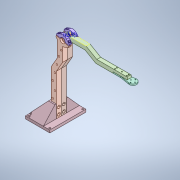
# Autodesk Inventor part: Луч
Saved by Autodesk Inventor 2021.2 (Build 252289000, 289)
## iProperties
Created: 2024-10-23
Part Number: Луч
Material: Типовые
Document SubType Name: Modeling
Designer: barko
Density: 1 g/cm^3
Appearance: По умолчанию
Author: barko
Autodesk Inventor part; units mm, degrees
ref_plane "XZ Plane" through (0, 0, 0) normal (0, 1, 0) x (-1, 0, 0)
ref_plane "XY Plane" through (0, 0, 0) normal (0, 0, 1) x (1, 0, 0)
sketch "Эскиз1" plane through (0, 0, 0) normal (0, 0, 1) x (1, 0, 0)
  circle A0 centre (0, 0) radius 5 construction
  line L0 (381, 7) -> (127, 7) construction
  line L1 (127, 7) -> (127, 17) construction
  line L2 (127, 17) -> (381, 17) construction
  line L3 (381, 17) -> (381, 7) construction
  line L4 (381, 7) -> (127, 17) construction
  line L5 (127, 7) -> (381, 17) construction
  arc A1 (0, 15) -> (14.8661, -2) centre (0, 0) ccw
  arc A2 (5.5, 0) -> (5.1235, -2) centre (0, 0) ccw
  line L6 (268, -19) -> (240, -19) construction
  line L7 (240, -19) -> (240, 7) construction
  line L8 (240, 7) -> (268, 7) construction
  line L9 (268, 7) -> (268, -19) construction
  line L10 (268, -19) -> (240, 7) construction
  line L11 (240, -19) -> (268, 7) construction
  line L12 (0, 15) -> (79.4308, 15)
  line L13 (79.4308, 15) -> (121, -9)
  line L14 (121, -9) -> (254, -9)
  line L15 (254, -9) -> (254, -24)
  line L16 (254, -24) -> (116.9808, -24)
  line L17 (116.9808, -24) -> (75.4115, 0)
  line L18 (75.4115, 0) -> (5.5, 0)
  line L19 (10, 15) -> (10, -15) construction
  line L20 (12.5, -6) -> (7.5, -6) construction
  line L21 (7.5, -6) -> (7.5, 13) construction
  line L22 (7.5, 13) -> (12.5, 13) construction
  line L23 (12.5, 13) -> (12.5, -6) construction
  line L24 (12.5, -6) -> (7.5, 13) construction
  line L25 (7.5, -6) -> (12.5, 13) construction
  line L26 (15, 13) -> (5, 13) construction
  line L27 (5, 13) -> (5, 16) construction
  line L28 (5, 16) -> (15, 16) construction
  line L29 (15, 16) -> (15, 13) construction
  line L30 (15, 13) -> (5, 16) construction
  line L31 (5, 13) -> (15, 16) construction
  line L32 (15, -15) -> (5, -15) construction
  line L33 (5, -15) -> (5, -6) construction
  line L34 (5, -6) -> (15, -6) construction
  line L35 (15, -6) -> (15, -15) construction
  line L36 (15, -15) -> (5, -6) construction
  line L37 (5, -15) -> (15, -6) construction
  line L38 (14.8661, -2) -> (5.1235, -2)
  line L39 (14.8661, -2) -> (15.8661, -2)
  line L40 (15.8661, -2) -> (15.8661, -12)
  line L41 (15.8661, -12) -> (9, -12)
  point P0 (254, 12)
  point P1 (254, -6)
  point P2 (254, -6)
  point P3 (254, 12)
  point P4 (10, 3.5)
  point P5 (10, 14.5)
  point P6 (10, -10.5)
  point P7 (10, -6)
  point P8 (10, 13)
  point P9 (13.7477, -6)
  dimension "d0" = 10
  dimension "d1" = 10
  dimension "d2" = 254
  dimension "d3" = 254
  dimension "d4" = 7
  dimension "d6" = 26
  dimension "d8" = 28
  dimension "d9" = 15
  dimension "d10" = 15
  dimension "d11" = 15
  dimension "d12" = 5
  dimension "d14" = 0.5
  dimension "d17" = 0
  dimension "d21" = 5
  dimension "d23" = 2
  dimension "d24" = 10
  dimension "d25" = 10
  dimension "d27" = 1
  dimension "d29" = 30
  dimension "d30" = 6
  dimension "d31" = 0
  dimension "d48" = 24
  dimension "d78" = 2
  dimension "d79" = 2
  dimension "d80" = 4
  dimension "d115" = 0
  dimension "d237" = 10
  dimension "d245" = 1
  constraints: 84 end point, 17 midpoint, 12 parallel, 10 horizontal, 7 perpendicular, 7 point on circle, 6 point on line, 3 centre point, 3 coincident, 2 vertical, 1 tangent, 1 vertical alignment
  measures "d0" diameter of A0
  measures "d1" distance of L0.end L1.end
  measures "d2" distance of L1.end L2.end
  measures "d3" horizontal distance of point (254, 12) point (0, 0)
  measures "d4" distance from line of point (0, 0) L0
  measures "d6" distance of L8.end L6.start
  measures "d8" distance of L6.start L6.end
  measures "d9" distance between parallel lines of L12 L18
  measures "d10" distance between parallel lines of L13 L17
  measures "d11" distance between parallel lines of L16 L14
  measures "d12" distance between parallel lines of L6 L16
  measures "d14" radial gap between concentric circles of A0 A2
  measures "d17" distance from line of point (0, 0) L18
  measures "d21" distance of L21.end L22.end
  measures "d23" distance between parallel lines of L12 L26
  measures "d24" distance of L32.start L32.end
  measures "d25" distance of L27.end L28.end
  measures "d27" distance between parallel lines of L12 L28
  measures "d29" angle of L12 L13
  measures "d30" distance from line of L1 L13.end
  measures "d31" distance from line of point (254, -6) L15
  measures "d48" distance between parallel lines of L18 L16
  measures "d78" distance between parallel lines of L18 L38
  measures "d79" distance edge to line of A2 L21
  measures "d80" distance between parallel lines of L38 L20
  measures "d115" distance edge to line of A1 L32
  measures "d237" distance of L39.end L40.end
  measures "d245" distance of L38.start L39.end
extrude "Выдавливание1" add sketch "Эскиз1" along normal mid plane 15
sketch "Эскиз2" plane through (116.9808, -24, 7.5) normal (0, -1, 0) x (1, 0, 0)
  circle A0 centre (137.0192, -7.5) radius 14
  circle A1 centre (137.0192, -7.5) radius 16
  line L0 (0, 0) -> (137.0192, 0) construction
  line L1 (137.0192, -15) -> (0, -15) construction
  line L2 (97.0192, 0) -> (134.7082, 6.3079)
  line L3 (4.0192, -15) -> (137.0192, -15) construction
  line L4 (97.0192, -15) -> (134.7082, -21.3079)
  line L5 (97.0192, 0) -> (97.0192, -15)
  line L6 (97.0192, 0) -> (67.0192, 0)
  line L7 (67.0192, 0) -> (67.0192, -15)
  line L8 (67.0192, -15) -> (97.0192, -15)
  point P0 (-116.9808, -7.5)
  point P1 (137.0192, -7.5)
  dimension "d34" = 28
  dimension "d35" = 2
  dimension "d40" = 40
  dimension "d75" = 30
  constraints: 12 end point, 4 point on line, 2 centre point, 2 coincident, 2 perpendicular, 2 point on circle, 2 tangent, 1 vertical
  measures "d34" diameter of A0
  measures "d35" radial gap between concentric circles of A0 A1
  measures "d40" horizontal distance of A0.centre L2.start
  measures "d75" distance between parallel lines of L5 L7
extrude "Выдавливание2" add sketch "Эскиз2" against normal blind 5 separate body contours A0 | A0 L4 A1 L2 | A1 L4 L5 L2 | L5 L8 L7 L6 picked at (121.8202, -8.6894)
extrude "Выдавливание3" cut sketch "Эскиз2" against normal up to surface (10 mm away) from surface at -5 contours A0 | A0 L2 A1 L4 | A0 L4 A1 L2 bodies 1
extrude "Выдавливание11" cut sketch "Эскиз2" against normal up to surface (5 mm away) from surface at 0 contours A0 | A0 L4 A1 L2 | A1 L4 L5 L2 | L5 L8 L7 L6 picked at (121.8202, -8.6894) bodies 1
sketch "Эскиз3" plane through (0, 0, 0) normal (0, 0, 1) x (1, 0, 0)
  line L0 (-250, -275) -> (250, -275) construction
  circle A0 centre (0, 0) radius 381 construction
  circle A1 centre (0, 0) radius 9.5 construction
  arc A2 (-9.9382, 1.11) -> (9.1617, -4.0078) centre (0, 0) ccw
  arc A3 (-19.6523, 3.7129) -> (18.8759, -6.6107) centre (0, 0) ccw
  line L1 (-20, 0) -> (-20, -7.0273) construction
  line L2 (0, -73.4115) -> (0, -20)
  line L3 (251.689, -24) -> (268, -24) construction
  line L4 (116.9808, -24) -> (75.4115, 0) construction
  circle A4 centre (0, 0) radius 75.4115 construction
  arc A5 (5.5, 0) -> (5.1235, -2) centre (0, 0) ccw construction
  line L5 (254, -24) -> (116.9808, -24) construction
  circle A6 centre (0, 0) radius 119.4173 construction
  circle A7 centre (0, 0) radius 269.0725 construction
  line L6 (0, -73.4115) -> (-24, -114.9808)
  line L7 (-24, -114.9808) -> (-24, -275)
  line L8 (-20, -68.0526) -> (-44, -109.6218)
  line L9 (-44, -109.6218) -> (-44, -275)
  line L10 (-44, -275) -> (-24, -275)
  line L11 (-19.6523, 3.7129) -> (18.8759, -6.6107)
  line L12 (-18.8759, 6.6107) -> (19.6523, -3.7129)
  line L13 (-533.4, 0) -> (533.4, 0) construction
  arc A8 (19.6523, -3.7129) -> (-18.8759, 6.6107) centre (0, 0) ccw
  arc A9 (-9.1617, 4.0078) -> (-9.9382, 1.11) centre (0, 0) ccw
  arc A10 (9.1617, -4.0078) -> (9.9382, -1.11) centre (0, 0) ccw
  arc A11 (9.9382, -1.11) -> (-9.1617, 4.0078) centre (0, 0) ccw
  circle A12 centre (0, 0) radius 6.5
  line L14 (-18.8759, 6.6107) -> (-23.7055, 7.9048)
  line L15 (-22.4114, 12.7344) -> (-16.5875, 11.1739)
  line L16 (-19.6523, 3.7129) -> (-24.482, 5.007)
  line L17 (-25.7761, 0.1774) -> (-19.9521, -1.3831)
  line L18 (-23.7055, 7.9048) -> (-22.4114, 12.7344)
  line L19 (-24.482, 5.007) -> (-25.7761, 0.1774)
  line L20 (-22.4114, 12.7344) -> (-7.2587, 18.6363)
  line L21 (-25.7761, 0.1774) -> (-15.6044, -12.5101)
  line L22 (19.6523, -3.7129) -> (24.482, -5.007)
  line L23 (24.482, -5.007) -> (25.7761, -0.1774)
  line L24 (25.7761, -0.1774) -> (15.6044, 12.5101)
  line L25 (25.7761, -0.1774) -> (19.9521, 1.3831)
  line L26 (18.8759, -6.6107) -> (23.7055, -7.9048)
  line L27 (23.7055, -7.9048) -> (22.4114, -12.7344)
  line L28 (22.4114, -12.7344) -> (16.5875, -11.1739)
  line L29 (22.4114, -12.7344) -> (7.2587, -18.6363)
  line L30 (-20, -7.0273) -> (-20, -68.0526)
  arc A13 (-20, -15) -> (0, -25) centre (0, 0) ccw
  arc A14 (0, 15) -> (9, -12) centre (0, 0) ccw construction
  line L31 (0, 0) -> (66.16, -375.2118) construction
  point P0 (0, -275)
  point P1 (0, -75.4115)
  point P2 (0, -119.4173)
  point P3 (5.7208, -3.0858)
  point P4 (-6.4973, 0.188)
  point P5 (-5.7208, 3.0858)
  point P6 (6.4973, -0.188)
  point P7 (-20, -1.3703)
  dimension "d107" = 381
  dimension "d108" = 538.145
  dimension "d43" = 275
  dimension "d44" = 500
  dimension "d45" = 19
  dimension "d46" = 0.5
  dimension "d47" = 20
  dimension "d49" = 30
  dimension "d50" = 24
  dimension "d53" = 20
  dimension "d54" = 20
  dimension "d56" = 3
  dimension "d57" = 1.5
  dimension "d58" = 15
  dimension "d59" = 3
  dimension "d93" = 5
  dimension "d94" = 5
  dimension "d95" = 5
  dimension "d102" = 5
  dimension "d105" = 80
  dimension "d246" = 2
  constraints: 56 end point, 20 point on circle, 10 centre point, 10 point on line, 9 coincident, 8 parallel, 7 perpendicular, 4 equal length, 4 vertical, 3 vertical alignment, 2 collinear, 2 horizontal, 2 tangent, 1 midpoint, 19 other
  measures "d43" distance from line of L0 point (0, 0)
  measures "d44" distance of L0.start L0.end
  measures "d45" diameter of A1
  measures "d46" radial gap between concentric circles of A1 A2
  measures "d47" distance between parallel lines of L2 L1
  measures "d49" angle of L2 L6
  measures "d50" distance between parallel lines of L2 L7
  measures "d53" distance between parallel lines of L6 L8
  measures "d54" distance between parallel lines of L7 L9
  measures "d56" distance between parallel lines of L12 L11
  measures "d57" distance from line of point (0, 0) L12
  measures "d58" angle of L13 L11
  measures "d59" radial gap between concentric circles of A12 A1
  measures "d93" distance between parallel lines of L15 L14
  measures "d94" distance between parallel lines of L17 L16
  measures "d95" distance of L12.start L14.end
  measures "d105" angle of L13 L31
  measures "d246" distance of A4.end L2.start
ref_plane "РабПлоскость1" through (0, 0, 9.5) normal (0, 0, 1) x (1, 0, 0)
extrude "Выдавливание12" add sketch "Эскиз3" along normal blind 3 from surface at 9.5 separate body contours L11 A12 A2 | A2 L11 A3
extrude "Выдавливание13" add sketch "Эскиз3" along normal blind 7 from surface at 12.5 contours A2 L11 A3 bodies 3
extrude "Выдавливание17" add sketch "Эскиз3" along normal up to surface (10 mm away) from surface at 9.5 contours A3 L17 L19 L16 | L26 L27 L28 A3 | A3 L21 L17 | L28 L29 A3 bodies 3
extrude "Выдавливание15" add sketch "Эскиз3" along normal up to surface (3 mm away) from surface at 9.5 separate body contours A11 L12 A12 | L12 A8 A11
extrude "Выдавливание16" add sketch "Эскиз3" along normal up to surface (7 mm away) from surface at 12.5 contours L12 A8 A11 bodies 4
extrude "Выдавливание18" add sketch "Эскиз3" along normal up to surface (10 mm away) from surface at 9.5 contours L14 L18 L15 A8 | A8 L25 L23 L22 | L15 L20 A8 | A8 L24 L25 bodies 4
extrude "Выдавливание19" add sketch "Эскиз3" along normal up to surface (10 mm away) from surface at 9.5 contours A3 L2 A13 L30 L21 | L2 L6 L7 L10 L9 L8 L30 A13 bodies 3
extrude "Выдавливание20" add sketch "Эскиз3" along normal up to surface (9.5 mm away) contours L2 L6 L7 L10 L9 L8 L30 A13 bodies 3
sketch "Эскиз4" plane through (0, 0, 0) normal (0, 0, 1) x (1, 0, 0)
  circle A0 centre (0, 0) radius 269.0725 construction
  circle A1 centre (0, 0) radius 119.4173 construction
  line L0 (184, -24) -> (116.9808, -24) construction
  line L1 (268, -24) -> (116.9808, -24) construction
  line L2 (116.9808, -24) -> (0, 0) construction
  arc A2 (5.5, 0) -> (5.1235, -2) centre (0, 0) ccw construction
  line L3 (-3.3219, -119.3711) -> (22.9023, -268.096) construction
  line L4 (-3.3219, -119.3711) -> (0, 0) construction
  line L5 (-44, -109.6218) -> (-44, -275) construction
  line L6 (-44, -275) -> (-24, -275) construction
  line L7 (-24, -275) -> (-24, -114.9808) construction
  line L8 (381, 7) -> (127, 7) construction
  line L9 (28.947, -123.855) -> (73.0536, -373.9962) construction
  arc A3 (28.947, -123.855) -> (127, 7) centre (0, 0) ccw construction
  line L10 (1, -275) -> (-94, -275)
  line L11 (-94, -275) -> (-94, -285)
  line L12 (-94, -285) -> (1, -285)
  line L13 (1, -285) -> (1, -275)
  line L14 (-44, -275) -> (-44, -109.6218) construction
  line L15 (-24, -275) -> (-44, -275) construction
  dimension "d109" = 168.406
  dimension "d110" = 0
  dimension "d112" = 149.6551
  dimension "d113" = 168.406
  dimension "d114" = 80
  dimension "d116" = 31
  dimension "d117" = 31
  dimension "d118" = 10
  dimension "d119" = 25
  dimension "d120" = 50
  constraints: 18 end point, 6 point on circle, 3 parallel, 1 centre point, 1 coincident, 1 collinear, 1 equal length, 1 horizontal, 1 perpendicular, 1 point on line
  measures "d109" angle of L2 L1
  measures "d110" distance between parallel lines of L0 L1
  measures "d112" radial gap between concentric circles of A1 A0
  measures "d113" angle of L4 L3
  measures "d114" angle of L2 L4
  measures "d116" distance between parallel lines of L0 L8
  measures "d117" distance between parallel lines of L3 L9
  measures "d118" distance of L12.end L10.start
  measures "d119" distance between parallel lines of L7 L13
  measures "d120" distance between parallel lines of L5 L11
ref_plane "РабПлоскость2" through (-44, -275, 69.5) normal (0, 0, 1) x (1, 0, 0)
extrude "Выдавливание24" add sketch "Эскиз4" along normal blind 70 separate body
ref_plane "РабПлоскость3" through (-94, -225, 0) normal (0, 1, 0) x (1, 0, 0)
sketch "Эскиз6" plane through (-94, -225, 0) normal (0, 1, 0) x (1, 0, 0)
  line L0 (103.1617, -19.5) -> (117.7055, -19.5) construction
  line L1 (84.0618, -19.5) -> (103.1617, -19.5) construction
  line L2 (69.518, -19.5) -> (84.0618, -19.5) construction
  line L3 (68.2239, -19.5) -> (69.518, -19.5) construction
  line L4 (74, -19.5) -> (68.2239, -19.5) construction
  line L5 (50, -19.5) -> (74, -19.5) construction
  line L6 (70, -19.5) -> (50, -19.5) construction
  line L7 (94, -19.5) -> (70, -19.5) construction
  line L8 (101.2587, -19.5) -> (94, -19.5) construction
  line L9 (116.4114, -19.5) -> (101.2587, -19.5) construction
  line L10 (117.7055, -19.5) -> (116.4114, -19.5) construction
  line L11 (50, 0) -> (50, -19.5) construction
  line L12 (50, 0) -> (50, -19.5) construction
  line L13 (70, 0) -> (94, 0) construction
  line L14 (50, 0) -> (70, 0) construction
  line L15 (74, 0) -> (50, 0) construction
  line L16 (94, 0) -> (74, 0) construction
  line L17 (70, 0) -> (70, -19.5) construction
  line L18 (70, 0) -> (70, -19.5) construction
  line L19 (95, 0) -> (95, -70) construction
  line L20 (95, 0) -> (0, 0) construction
  line L21 (0, 0) -> (0, -70) construction
  line L22 (95, 0) -> (0, 0) construction
  line L23 (49.5, 0) -> (49.5, -20)
  line L24 (49.5, -20) -> (70, -20)
  line L25 (70, 0) -> (70, -19.5) construction
  line L26 (70, -20) -> (70, 0)
  line L27 (70, 0) -> (49.5, 0)
  line L28 (49.5, 0) -> (44.5, 0)
  line L29 (44.5, 0) -> (44.5, -25)
  line L30 (44.5, -25) -> (70, -25)
  line L31 (70, -25) -> (70, -20)
  line L32 (95, -70) -> (0, -70) projected
  point P0 (94, 0)
  dimension "d136" = 0.5
  dimension "d137" = 0.5
  dimension "d148" = 5
  dimension "d149" = 5
  constraints: 16 end point, 4 perpendicular, 2 vertical, 1 collinear, 3 other
  measures "d136" distance between parallel lines of L11 L23
  measures "d137" distance between parallel lines of L6 L24
  measures "d148" distance between parallel lines of L23 L29
  measures "d149" distance between parallel lines of L24 L30
sketch "Эскиз7" plane through (-94, -275, 0) normal (0, 1, 0) x (1, 0, 0)
  line L0 (95, 0) -> (0, 0) construction
  line L1 (70, 0) -> (70, -19.5) construction
  line L2 (0, 0) -> (70, 0)
  line L3 (70, 0) -> (70, -70)
  line L4 (0, 0) -> (0, -70) construction
  line L5 (0, 0) -> (0, -70) construction
  line L6 (0, 0) -> (0, -70)
  line L7 (0, -70) -> (70, -70)
  line L8 (95, -70) -> (0, -70) construction
  point P0 (94, 0)
  dimension "d191" = 0
  constraints: 8 end point, 2 perpendicular, 1 horizontal, 1 vertical
  measures "d191" distance between parallel lines of L8 L7
loft "Лофт1" add profiles "Эскиз7", "Эскиз6" bodies 5
extrude "Выдавливание25" cut sketch "Эскиз6" against normal up to surface (50 mm away) contours L27 L26 L24 L23 bodies 5
ref_plane "РабПлоскость5" through (-49.5, -225, 25) normal (1, 0, 0) x (0, 1, 0)
sketch "Эскиз9" plane through (-24, -225, 25) normal (1, 0, 0) x (0, 1, 0)
  line L0 (-8.9378, -15.25) -> (-11.9689, -20.5)
  line L1 (-11.9689, -20.5) -> (-18.0311, -20.5)
  line L2 (-18.0311, -20.5) -> (-21.0622, -15.25)
  line L3 (-21.0622, -15.25) -> (-18.0311, -10)
  line L4 (-18.0311, -10) -> (-11.9689, -10)
  line L5 (-11.9689, -10) -> (-8.9378, -15.25)
  circle A0 centre (-15, -15.25) radius 5.25 construction
  line L6 (-50, -5.5) -> (115.3782, -5.5) construction
  line L7 (115.3782, -25) -> (-50, -25) construction
  line L8 (0, 0) -> (0, -25) construction
  line L9 (-11.2472, -15.25) -> (-13.1236, -18.5)
  line L10 (-13.1236, -18.5) -> (-16.8764, -18.5)
  line L11 (-16.8764, -18.5) -> (-18.7528, -15.25)
  line L12 (-18.7528, -15.25) -> (-16.8764, -12)
  line L13 (-16.8764, -12) -> (-13.1236, -12)
  line L14 (-13.1236, -12) -> (-11.2472, -15.25)
  circle A1 centre (-15, -15.25) radius 3.25 construction
  line L15 (0, -21.8122) -> (-15, -21.8122)
  arc A2 (-15, -8.6878) -> (-15, -21.8122) centre (-15, -15.25) ccw
  line L16 (-15, -8.6878) -> (0, -8.6878)
  line L17 (0, -21.8122) -> (0, -8.6878)
  circle A3 centre (-15, -15.25) radius 6.0622 construction
  line L18 (-15, -15.25) -> (-40, -15.25)
  line L19 (-36.2472, -15.25) -> (-38.1236, -18.5)
  circle A4 centre (-40, -15.25) radius 3.25 construction
  line L20 (-41.8764, -18.5) -> (-43.7528, -15.25)
  line L21 (-33.9378, -15.25) -> (-36.9689, -20.5)
  line L22 (-36.9689, -20.5) -> (-43.0311, -20.5)
  circle A5 centre (-40, -15.25) radius 5.25 construction
  line L23 (-43.0311, -20.5) -> (-46.0622, -15.25)
  circle A6 centre (-40, -15.25) radius 6.0622 construction
  line L24 (-43.0311, -10) -> (-36.9689, -10)
  line L25 (-36.9689, -10) -> (-33.9378, -15.25)
  line L26 (-41.8764, -12) -> (-38.1236, -12)
  line L27 (-38.1236, -12) -> (-36.2472, -15.25)
  line L28 (-46.0622, -15.25) -> (-43.0311, -10)
  line L29 (-38.1236, -18.5) -> (-41.8764, -18.5)
  line L30 (-43.7528, -15.25) -> (-41.8764, -12)
  line L31 (-15, -8.6878) -> (-40, -8.6878)
  line L32 (110.0192, -5.5) -> (-50, -5.5) construction
  line L33 (-40, -21.8122) -> (-15, -21.8122)
  arc A7 (-40, -8.6878) -> (-40, -21.8122) centre (-40, -15.25) ccw
  point P0 (225, -25)
  dimension "d145" = 10.5
  dimension "d146" = 19.5
  dimension "d147" = 9.75
  dimension "d152" = 15
  dimension "d153" = 6.5
  dimension "d161" = 0.5
  dimension "d166" = 25
  constraints: 60 end point, 12 coincident, 7 tangent, 6 centre point, 6 horizontal, 5 point on circle, 2 horizontal alignment, 2 parallel, 2 point on line, 1 collinear, 1 perpendicular, 62 other
  measures "d145" distance between parallel lines of L4 L1
  measures "d146" distance between parallel lines of L6 L7
  measures "d147" distance from line of L7 point (-15, -15.25)
  measures "d152" distance from line of point (-15, -15.25) L8
  measures "d153" diameter of A1
  measures "d166" distance of L9.start L19.start
extrude "Выдавливание27" cut sketch "Эскиз9" against normal blind 69.5 contours L9 L10 L11 L12 L13 L14 | L19 L29 L20 L30 L26 L27 bodies 3 5
extrude "Выдавливание28" cut sketch "Эскиз9" against normal blind 7 from surface at 0 contours L0 L1 L2 L3 L4 L5 | L19 L29 L20 L30 L26 L27 | L21 L22 L23 L28 L24 L25 bodies 3
ref_plane "РабПлоскость6" through (-55.5, -225, 25) normal (1, 0, 0) x (0, 1, 0)
ref_plane "РабПлоскость7" through (-75.5, -225, 25) normal (1, 0, 0) x (0, 1, 0)
extrude "Выдавливание26" cut sketch "Эскиз9" along normal blind 6 from surface at -31.5 contours L0 L1 L2 L3 L4 L5 | L9 L10 L11 L12 L13 L14 bodies 5
extrude "Выдавливание29" cut sketch "Эскиз9" against normal up to surface (38.5 mm away) from surface at -31.5 contours L0 L1 L2 L3 L4 L5 | L9 L10 L11 L12 L13 L14 | L15 A2 L16 L17 bodies 5
extrude "Выдавливание31" cut sketch "Эскиз9" along normal blind 5 from surface at -51.5 contours L21 L22 L23 L28 L24 L25 bodies 5
extrude "Выдавливание32" cut sketch "Эскиз9" against normal up to surface (18.5 mm away) from surface at -51.5 contours L15 A2 L16 L17 | L33 A7 L31 A2 | L19 L29 L20 L30 L26 L27 | L21 L22 L23 L28 L24 L25 bodies 5
sketch "Эскиз11" plane through (1, -275, 70) normal (0, 1, 0) x (1, 0, 0)
  line L0 (0, 70) -> (0, 0) construction
  line L1 (-95, 0) -> (0, 0) construction
  line L2 (0, 0) -> (-25, 0) construction
  line L3 (-25, 0) -> (-95, 0) construction
  line L4 (-95, 70) -> (-95, 0) construction
  line L5 (-95, 70) -> (-95, 0) construction
  line L6 (-95, 0) -> (0, 0) construction
  line L7 (-95, 0) -> (-95, 14.75)
  line L8 (-95, 70) -> (-95, 0) construction
  line L9 (-95, 14.75) -> (-88.75, 14.75)
  arc A0 (-80.25, 6.25) -> (-88.75, 14.75) centre (-88.75, 6.25) ccw
  line L10 (-80.25, 6.25) -> (-80.25, 0)
  line L11 (-95, 0) -> (-80.25, 0)
  circle A1 centre (-6.25, 6.25) radius 3.25
  circle A2 centre (-88.75, 6.25) radius 3.25
  circle A3 centre (-88.75, 6.25) radius 7.5 construction
  circle A4 centre (-88.75, 6.25) radius 5.5 construction
  point P0 (-1, 70)
  dimension "d196" = 6.5
  dimension "d197" = 3
  dimension "d199" = 3
  dimension "d200" = 3
  dimension "d201" = 3
  dimension "d202" = 11
  dimension "d203" = 15
  dimension "d204" = 1
  constraints: 8 end point, 5 centre point, 3 coincident, 2 point on circle, 2 point on line, 2 tangent, 1 collinear, 1 equal radius, 1 horizontal, 1 perpendicular
  measures "d196" diameter of A2
  measures "d197" distance edge to line of A2 L1
  measures "d199" distance edge to line of A1 L1
  measures "d200" distance edge to line of A1 L0
  measures "d201" distance edge to line of A2 L4
  measures "d202" diameter of A4
  measures "d203" diameter of A3
  measures "d204" radial gap between concentric circles of A3 A0
extrude "Выдавливание35" cut sketch "Эскиз11" against normal through all contours A1 | A2 bodies 5
extrude "Выдавливание36" cut sketch "Эскиз11" along normal up to next contours L7 L9 A0 L10 L11 | A2 bodies 5
ref_plane "РабПлоскость8" through (-6.1091, 1.6369, 9.5) normal (-0.258819, -0.9659258, 0) x (0.9659258, -0.258819, 0)
sketch "Эскиз12" plane through (-6.1091, 1.6369, 9.5) normal (-0.258819, -0.9659258, 0) x (0.9659258, -0.258819, 0)
  line L0 (-3.5623, 3) -> (-3.5623, 10) construction
  line L1 (-3.5623, 3) -> (-3.5623, 10) construction
  line L2 (16.2114, 3) -> (16.2114, 10) construction
  line L3 (16.2114, 10) -> (16.2114, 3) construction
  line L4 (-18.6191, 0) -> (-18.6191, 10) construction
  line L5 (31.2682, 0) -> (31.2682, 10) construction
  circle A0 centre (26.0182, 5) radius 2.25 construction
  circle A1 centre (-13.3691, 5) radius 2.25 construction
  line L6 (-5.5102, 10) -> (18.1593, 10) construction
  line L7 (-5.5102, 0) -> (18.1593, 0) construction
  line L8 (-18.6191, 0) -> (-5.5102, 0) construction
  line L9 (26.0182, 0.8431) -> (22.4182, 2.9215)
  line L10 (22.4182, 2.9215) -> (22.4182, 7.0785)
  line L11 (22.4182, 7.0785) -> (26.0182, 9.1569)
  line L12 (26.0182, 9.1569) -> (29.6182, 7.0785)
  line L13 (29.6182, 7.0785) -> (29.6182, 2.9215)
  line L14 (29.6182, 2.9215) -> (26.0182, 0.8431)
  line L15 (-13.3691, 0.8431) -> (-16.9691, 2.9215)
  line L16 (-16.9691, 2.9215) -> (-16.9691, 7.0785)
  line L17 (-16.9691, 7.0785) -> (-13.3691, 9.1569)
  line L18 (-13.3691, 9.1569) -> (-9.7691, 7.0785)
  line L19 (-9.7691, 7.0785) -> (-9.7691, 2.9215)
  line L20 (-9.7691, 2.9215) -> (-13.3691, 0.8431)
  circle A2 centre (-13.3691, 5) radius 4.1569 construction
  circle A3 centre (26.0182, 5) radius 4.1569 construction
  line L21 (26.0182, 2.4019) -> (23.7682, 3.701)
  line L22 (23.7682, 3.701) -> (23.7682, 6.299)
  line L23 (23.7682, 6.299) -> (26.0182, 7.5981)
  line L24 (26.0182, 7.5981) -> (28.2682, 6.299)
  line L25 (28.2682, 6.299) -> (28.2682, 3.701)
  line L26 (28.2682, 3.701) -> (26.0182, 2.4019)
  line L27 (-13.3691, 2.4019) -> (-15.6191, 3.701)
  line L28 (-15.6191, 3.701) -> (-15.6191, 6.299)
  line L29 (-15.6191, 6.299) -> (-13.3691, 7.5981)
  line L30 (-13.3691, 7.5981) -> (-11.1191, 6.299)
  line L31 (-11.1191, 6.299) -> (-11.1191, 3.701)
  line L32 (-11.1191, 3.701) -> (-13.3691, 2.4019)
  line L33 (-18.6191, 0) -> (-18.6191, 10) construction
  line L34 (-11.1752, 0) -> (-18.6191, 0) construction
  line L35 (31.2682, 0) -> (31.2682, 10) construction
  line L36 (16.2114, 10) -> (31.2682, 10) construction
  point P0 (6.3246, -9.5)
  dimension "d303" = 8.3138
  dimension "d304" = 8.3138
  dimension "d209" = 4.5
  dimension "d210" = 4.5
  dimension "d211" = 10
  dimension "d212" = 5
  dimension "d213" = 5
  dimension "d215" = 3
  dimension "d218" = 3
  dimension "d306" = 7.2
  constraints: 48 end point, 6 coincident, 4 parallel, 2 centre point, 2 tangent, 58 other
  measures "d209" diameter of A0
  measures "d210" diameter of A1
  measures "d211" distance between parallel lines of L6 L7
  measures "d212" distance from line of A0.centre L7
  measures "d213" distance from line of A1.centre L8
  measures "d215" distance edge to line of A0 L5
  measures "d218" distance edge to line of A1 L4
  measures "d306" distance between parallel lines of L19 L16
ref_plane "РабПлоскость9" through (-8.1796, -6.0905, 9.5) normal (-0.258819, -0.9659258, 0) x (0.9659258, -0.258819, 0)
extrude "Выдавливание39" cut sketch "Эскиз12" along normal blind 23 from surface at 8 contours L9 L10 L11 L12 L13 L14 | L15 L16 L17 L18 L19 L20 | L21 L22 L23 L24 L25 L26 | L27 L28 L29 L30 L31 L32 bodies 3
extrude "Выдавливание38" cut sketch "Эскиз12" along normal blind 14 contours L21 L22 L23 L24 L25 L26 | L27 L28 L29 L30 L31 L32 bodies 3
extrude "Выдавливание50" cut sketch "Эскиз12" against normal blind 33 contours L21 L22 L23 L24 L25 L26 | L27 L28 L29 L30 L31 L32 bodies 4
ref_plane "РабПлоскость10" through (-4.815, 6.4665, 9.5) normal (-0.258819, -0.9659258, 0) x (0.9659258, -0.258819, 0)
extrude "Выдавливание51" cut sketch "Эскиз12" against normal blind 33 from surface at -5 contours L9 L10 L11 L12 L13 L14 | L15 L16 L17 L18 L19 L20 | L21 L22 L23 L24 L25 L26 | L27 L28 L29 L30 L31 L32 bodies 4
sketch "Эскиз13" plane through (0, 15, 7.5) normal (0, 1, 0) x (1, 0, 0)
  line L0 (0, 0) -> (0, 15) construction
  line L1 (79.4308, 0) -> (0, 0) construction
  line L2 (79.4308, 15) -> (79.4308, 0) construction
  line L3 (0, 15) -> (79.4308, 15) construction
  line L4 (5.5, 15) -> (5.5, 0) construction
  circle A0 centre (9.05, 7.5) radius 2.05 construction
  line L5 (9.05, 3.3431) -> (5.45, 5.4215)
  line L6 (5.45, 5.4215) -> (5.45, 9.5785)
  line L7 (5.45, 9.5785) -> (9.05, 11.6569)
  line L8 (9.05, 11.6569) -> (12.65, 9.5785)
  line L9 (12.65, 9.5785) -> (12.65, 5.4215)
  line L10 (12.65, 5.4215) -> (9.05, 3.3431)
  line L11 (9.05, 5.1329) -> (7, 6.3164)
  line L12 (7, 6.3164) -> (7, 8.6836)
  line L13 (7, 8.6836) -> (9.05, 9.8671)
  line L14 (9.05, 9.8671) -> (11.1, 8.6836)
  line L15 (11.1, 8.6836) -> (11.1, 6.3164)
  line L16 (11.1, 6.3164) -> (9.05, 5.1329)
  line L17 (0, 15) -> (79.4308, 15) construction
  line L18 (15.8661, 15) -> (15.8661, 0) construction
  point P0 (0, 7.5)
  dimension "d226" = 4.1
  dimension "d227" = 5.45
  dimension "d228" = 5.45
  dimension "d229" = 7.2
  dimension "d391" = 1.5
  constraints: 24 end point, 2 coincident, 2 vertical, 1 centre point, 1 tangent, 26 other
  measures "d226" diameter of A0
  measures "d227" distance edge to line of A0 L1
  measures "d228" distance edge to line of A0 L3
  measures "d229" distance between parallel lines of L6 L9
  measures "d391" distance between parallel lines of L12 L4
extrude "Выдавливание40" cut sketch "Эскиз13" against normal blind 32 contours L11 L12 L13 L14 L15 L16 bodies 1
extrude "Выдавливание43" cut sketch "Эскиз13" against normal blind 5 bodies 1
ref_plane "РабПлоскость11" through (5.1235, -8, 7.5) normal (0, 1, 0) x (1, 0, 0)
extrude "Выдавливание44" cut sketch "Эскиз13" along normal up to surface (4 mm away) from surface at -27 contours L5 L6 L7 L8 L9 L10 | L11 L12 L13 L14 L15 L16 bodies 1
extrude "Выдавливание53" cut sketch "Эскиз13" against normal blind 10 from surface at -27 contours L5 L6 L7 L8 L9 L10 | L11 L12 L13 L14 L15 L16 bodies 1
mirror "Зеркальное отражение4" about plane through (0, 0, 0) normal (0, 0, 1) bodies 5
mirror "Зеркальное отражение5" about plane through (0, 0, 0) normal (0, 0, 1) bodies 3 4 separate body
sketch "Эскиз14" plane through (-44, -275, 19.5) normal (0, 0, 1) x (1, 0, 0)
  line L0 (0, 0) -> (0, 165.3782) construction
  line L1 (20, 160.0192) -> (20, 0) construction
  line L2 (24, 206.9474) -> (24, 267.9727) construction
  line L3 (0, 165.3782) -> (24, 206.9474) construction
  line L4 (0, 165.3782) -> (20, 160.0192) construction
  line L5 (24, 206.9474) -> (44, 201.5885) construction
  line L6 (24, 240) -> (52.5, 240) construction
  arc A0 (24, 260) -> (44, 250) centre (44, 275) ccw construction
  circle A1 centre (38.25, 240) radius 3.25
  circle A2 centre (38.25, 240) radius 1.75
  line L7 (44, 255) -> (44, 201.5885) construction
  line L8 (44, 201.5885) -> (20, 160.0192) construction
  line L9 (13, 31.2472) -> (0, 31.2472) construction
  line L10 (13, 13.7528) -> (0, 13.7528) construction
  line L11 (38.25, 243.2909) -> (41.1, 241.6454)
  line L12 (41.1, 241.6454) -> (41.1, 238.3546)
  line L13 (41.1, 238.3546) -> (38.25, 236.7091)
  line L14 (38.25, 236.7091) -> (35.4, 238.3546)
  line L15 (35.4, 238.3546) -> (35.4, 241.6454)
  line L16 (35.4, 241.6454) -> (38.25, 243.2909)
  point P0 (29.75, 215)
  point P1 (14.25, 151.9667)
  point P2 (5.75, 121.9667)
  point P3 (14.25, 91.9667)
  point P4 (5.75, 61.9667)
  point P5 (22, 183.4833)
  point P6 (44, 244.8338)
  dimension "d257" = 20
  dimension "d259" = 5.75
  dimension "d260" = 10
  dimension "d261" = 10
  dimension "d263" = 46.3644
  dimension "d264" = 23.1822
  dimension "d265" = 9.2664
  dimension "d266" = 9.2664
  dimension "d273" = 6.5
  dimension "d274" = 3.5
  dimension "d276" = 25
  dimension "d278" = 4
  dimension "d279" = 5.75
  dimension "d280" = 5.75
  dimension "d281" = 5.75
  dimension "d282" = 5.75
  dimension "d283" = 30
  dimension "d284" = 30
  dimension "d285" = 30
  dimension "d296" = 5.75
  dimension "d297" = 20
  dimension "d298" = 5.7
  constraints: 25 end point, 3 coincident, 2 centre point, 1 horizontal, 1 midpoint, 1 point on line, 1 vertical, 13 other
  measures "d257" distance between parallel lines of L0 L1
  measures "d259" distance from line of L2 point (29.75, 215)
  measures "d260" distance from line of L3 point (22, 183.483)
  measures "d261" distance from line of A0.end L6
  measures "d263" distance between parallel lines of L5 L4
  measures "d264" distance from line of point (22, 183.483) L5
  measures "d265" distance from line of L5 point (29.75, 215)
  measures "d266" distance from line of L4 point (14.25, 151.967)
  measures "d273" diameter of A1
  measures "d274" diameter of A2
  measures "d276" vertical distance of A1.centre point (29.75, 215)
  measures "d278" distance edge to line of A2 L7
  measures "d279" distance from line of point (14.25, 151.967) L1
  measures "d280" distance from line of L0 point (5.75, 121.967)
  measures "d281" distance from line of L1 point (14.25, 91.967)
  measures "d282" distance from line of L0 point (5.75, 61.967)
  measures "d283" vertical distance of point (5.75, 121.967) point (14.25, 151.967)
  measures "d284" vertical distance of point (5.75, 121.967) point (14.25, 91.967)
  measures "d285" vertical distance of point (5.75, 61.967) point (14.25, 91.967)
  measures "d296" distance from line of L7 A1.centre
  measures "d297" distance between parallel lines of L3 L8
  measures "d298" distance between parallel lines of L15 L12
extrude "Выдавливание45" cut sketch "Эскиз14" against normal up to surface (39 mm away) contours A2 bodies 3 6
extrude "Выдавливание48" cut sketch "Эскиз14" against normal blind 8 contours A1 L12 | L12 A1 L13 L14 L15 L16 L11 | L11 A1 | A1 L13 | L16 A1 | A1 L14 | L15 A1 bodies 3
extrude "Выдавливание49" cut sketch "Эскиз14" along normal blind 8 from surface at -39 contours L12 A1 L13 L14 L15 L16 L11 | A1 L11 L12 | L12 L13 A1 | A1 L16 L11 | L13 L14 A1 | A1 L15 L16 | L14 L15 A1 | A2 bodies 3 6
pattern_sketch "Массив по эскизу1" of "Выдавливание45", "Выдавливание49", "Выдавливание48" from (-5.75, -35, 19.5) bodies 3 6 copies at (-14.25, -60, 19.5) at (-29.75, -123.0333, 19.5) at (-38.25, -153.0333, 19.5) at (-29.75, -183.0333, 19.5) at (-38.25, -213.0333, 19.5) at (-22, -91.5167, 19.5)
sketch "Эскиз15" plane through (116.9808, -24, 7.5) normal (0, -1, 0) x (1, 0, 0)
  arc A0 (122.8859, 0) -> (122.8859, -15) centre (137.0192, -7.5) ccw construction
  arc A1 (122.8859, 0) -> (122.8859, -15) centre (137.0192, -7.5) ccw construction
  arc A2 (134.7082, -21.3079) -> (134.7082, 6.3079) centre (137.0192, -7.5) ccw construction
  line L0 (134.7082, 6.3079) -> (97.0192, 0) construction
  line L1 (97.0192, 0) -> (67.0192, 0) construction
  line L2 (67.0192, 0) -> (67.0192, -15) construction
  line L3 (67.0192, -15) -> (97.0192, -15) construction
  line L4 (97.0192, -15) -> (134.7082, -21.3079) construction
  line L5 (117.0192, -4) -> (71.0192, -4) construction
  line L6 (71.0192, -4) -> (71.0192, -11) construction
  line L7 (71.0192, -11) -> (117.0192, -11) construction
  line L8 (117.0192, -11) -> (117.0192, -4) construction
  line L9 (117.0192, -4) -> (71.0192, -11) construction
  line L10 (71.0192, -4) -> (117.0192, -11) construction
  circle A3 centre (71.0192, -11) radius 2 construction
  line L11 (71.0192, -13) -> (69.2872, -12)
  line L12 (69.2872, -12) -> (69.2872, -10)
  line L13 (69.2872, -10) -> (71.0192, -9)
  line L14 (71.0192, -9) -> (72.7513, -10)
  line L15 (72.7513, -10) -> (72.7513, -12)
  line L16 (72.7513, -12) -> (71.0192, -13)
  point P0 (-116.9808, -7.5)
  point P1 (94.0192, -7.5)
  point P2 (94.0192, -7.5)
  dimension "d322" = 4
  dimension "d318" = 4
  dimension "d319" = 4
  dimension "d320" = 4
  dimension "d321" = 4
  constraints: 24 end point, 7 coincident, 2 midpoint, 2 parallel, 1 horizontal, 1 perpendicular, 1 point on line, 1 vertical alignment, 15 other
  measures "d318" distance between parallel lines of L2 L6
  measures "d319" distance edge to line of A0 L8
  measures "d320" distance between parallel lines of L3 L7
  measures "d321" distance between parallel lines of L1 L5
extrude "Выдавливание52" cut sketch "Эскиз15" against normal through all bodies 1
pattern_sketch "Массив по эскизу2" of "Выдавливание52" from (188, -24, -3.5) bodies 1 copies at (234, -24, -3.5) at (234, -24, 3.5) at (211, -24, 0) at (188, -24, 3.5)
hole "Отверстие1" at (234, -24, -3.5) at (234, -24, 3.5) at (211, -24, 0) at (188, -24, 3.5) at (188, -24, -3.5) direction (0, 1, 0) diameter 3.4 end through all countersink diameter 6.6 countersink angle 90 bodies 2 clearance for "с потайной головкой ГОСТ 12876-67" size "M3" standard "ГОСТ"
sketch "Эскиз16" plane through (116.9808, -24, 7.5) normal (0, -1, 0) x (1, 0, 0)
  arc A0 (134.7082, -21.3079) -> (134.7082, 6.3079) centre (137.0192, -7.5) ccw construction
  line L0 (117.8155, -83.4683) -> (152.5625, -83.4683) construction
  line L1 (152.5625, -83.4683) -> (152.5625, -114.3585) construction
  line L2 (152.5625, -114.3585) -> (117.8155, -114.3585) construction
  line L3 (117.8155, -114.3585) -> (117.8155, -83.4683) construction
  arc A1 (128.4887, -104.7382) -> (127.1712, -99.0353) centre (126.8158, -102.121) ccw construction
  arc A2 (143.5579, -94.1085) -> (145.1461, -99.8294) centre (145.2615, -96.7165) ccw construction
  circle A3 centre (136.0822, -99.3963) radius 4.3502 construction
  circle A4 centre (143.0469, -103.233) radius 1.6875
  circle A5 centre (131.4452, -107.7401) radius 1.6875
  circle A6 centre (129.0288, -95.5762) radius 1.6875
  circle A7 centre (140.6306, -91.0691) radius 1.6875
  line L4 (143.0469, -103.233) -> (140.6306, -91.0691)
  line L5 (140.6306, -91.0691) -> (129.0288, -95.5762)
  line L6 (129.0288, -95.5762) -> (131.4452, -107.7401)
  line L7 (131.4452, -107.7401) -> (143.0469, -103.233)
  line L8 (137.0541, 2.0169) -> (129.0328, -7.5) construction
  line L9 (129.0328, -7.5) -> (136.9843, -17.0169) construction
  line L10 (136.9843, -17.0169) -> (145.0057, -7.5) construction
  line L11 (145.0057, -7.5) -> (137.0541, 2.0169) construction
  line L12 (145.0057, -7.5) -> (129.0328, -7.5) construction
  line L13 (137.0541, 2.0169) -> (136.9843, -17.0169) construction
  point P0 (-116.9808, -7.5)
  dimension "d338" = 13
  dimension "d352" = 3.375
  dimension "d363" = 12.4464
  dimension "d364" = 12.4016
  dimension "d365" = 12.4464
  dimension "d366" = 12.4016
  dimension "d367" = 15.9729
  dimension "d368" = 12.4464
  dimension "d369" = 12.4016
  dimension "d370" = 15.9729
  constraints: 20 end point, 7 centre point, 4 coincident, 4 parallel, 4 point on circle, 3 equal radius, 2 point on line, 1 horizontal, 1 midpoint, 2 other
  measures "d352" diameter of A4
  measures "d363" distance of L6.end L4.start
  measures "d364" distance of L5.end L6.end
  measures "d365" distance of L4.end L5.end
  measures "d366" distance of L4.start L4.end
  measures "d367" distance of L5.end L4.start
  measures "d368" distance of L8.start L8.end
  measures "d369" distance of L10.end L11.end
  measures "d370" distance of L8.end L10.end
hole "Отверстие2" at (246.0135, -24, 0) at (261.9865, -24, 0) at (254.0349, -24, 9.5169) at (253.9651, -24, -9.5169) direction (0, 1, 0) diameter 3.4 end through all countersink diameter 6.6 countersink angle 90 bodies 2 clearance for "с потайной головкой ГОСТ 12876-67" size "M3" standard "ГОСТ"
equation "\"d0\" = shaft_beam_diameter"
equation "\"d1\" = blade_height"
equation "\"d2\" = 2 * blade_radius"
equation "\"d3\" = beam_length"
equation "\"d8\" = motor_diameter"
equation "\"blade_radius\" = 127"
equation "\"blade_height\" = 10"
equation "\"bearing_inner\" = 7"
equation "\"bearing_outer\" = 19"
equation "\"bearing_width\" = 6"
equation "\"beam_length\" = 254"
equation "\"motor_height\" = 24"
equation "\"motor_diameter\" = 28"
equation "\"shaft_beam_diameter\" = 10"
equation "\"motor_blade_offset\" = 2"
